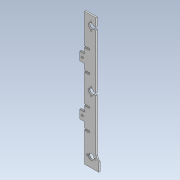
# Autodesk Inventor part: chassis_1_1_3
Saved by Autodesk Inventor 2022 (Build 260153000, 153)
## iProperties
Created: 2023-04-21
Part Number: chassis_1_1_3
Material: 一般
Document SubType Name: Modeling
Designer: JOU
Density: 1 g/cm^3
Appearance: 預設
Author: JOU
Autodesk Inventor part; units mm, degrees
ref_plane "YZ Plane" through (0, 0, 0) normal (1, 0, 0) x (0, 1, 0)
ref_plane "XZ Plane" through (0, 0, 0) normal (0, 1, 0) x (-1, 0, 0)
ref_plane "XY Plane" through (0, 0, 0) normal (0, 0, 1) x (1, 0, 0)
sketch "草圖1" plane through (0, 0, 0) normal (0, 0, 1) x (1, 0, 0)
  line L0 (-6, 142.5) -> (-10.5456, 142.5)
  arc A0 (-10.5456, 147.5) -> (-10.5456, 142.5) centre (-16, 145) ccw
  line L1 (-10.5456, 147.5) -> (-6, 147.5)
  circle A1 centre (-16, 153.5) radius 1.5
  circle A2 centre (-16, 136.5) radius 1.5
  circle A3 centre (-16, 275) radius 1.5
  circle A4 centre (-16, 258) radius 1.5
  circle A5 centre (-16, 23.5) radius 6
  circle A6 centre (-24.5, 23.5) radius 1.5
  circle A7 centre (-7.5, 23.5) radius 1.5
  line L2 (-6, 3) -> (-6, 16)
  line L3 (-6, 31) -> (-6, 142.5)
  arc A8 (-6, 16) -> (-6, 31) centre (-16, 23.5) ccw
  line L4 (-28.5, 3) -> (-28.5, 287)
  arc A9 (-10.546, 269.0008) -> (-10.546, 263.9992) centre (-16, 266.5) ccw
  line L5 (-28.5, 3) -> (-6, 3)
  line L6 (-6, 287) -> (-28.5, 287)
  line L7 (-6, 269.0008) -> (-10.546, 269.0008)
  line L8 (-10.546, 263.9992) -> (-6, 263.9992)
  line L9 (-6, 147.5) -> (-6, 263.9992)
  line L10 (-6, 269.0008) -> (-6, 287)
  circle A10 centre (-16, 23.5) radius 12.5 construction
  line L11 (-6, 72.05) -> (-6, 75)
  line L12 (-19.5, 70) -> (-19.5, 67.05)
  line L13 (-19.5, 112.05) -> (-19.5, 115)
  line L14 (-6, 110) -> (-6, 107.05)
  line L15 (-6, 182.95) -> (-6, 180)
  line L16 (-6, 217.95) -> (-6, 215)
  line L17 (-19.5, 67.05) -> (-28.5, 67.05)
  line L18 (-28.5, 67.05) -> (-28.5, 70)
  line L19 (-28.5, 70) -> (-19.5, 70)
  line L20 (-19.5, 70) -> (-19.5, 67.05)
  line L21 (-19.5, 112.05) -> (-28.5, 112.05)
  line L22 (-28.5, 112.05) -> (-28.5, 115)
  line L23 (-28.5, 115) -> (-19.5, 115)
  line L24 (-19.5, 115) -> (-19.5, 112.05)
  line L25 (-19.5, 175) -> (-28.5, 175)
  line L26 (-28.5, 175) -> (-28.5, 177.95)
  line L27 (-28.5, 177.95) -> (-19.5, 177.95)
  line L28 (-19.5, 177.95) -> (-19.5, 175)
  line L29 (-28.5, 220) -> (-19.5, 220)
  line L30 (-19.5, 220) -> (-19.5, 222.95)
  line L31 (-19.5, 222.95) -> (-28.5, 222.95)
  line L32 (-28.5, 222.95) -> (-28.5, 220)
  line L33 (-6, 3) -> (-3.5, 3)
  line L34 (-3.5, 3) -> (-3.5, 23.5)
  line L35 (-3.5, 23.5) -> (-6, 23.5)
  line L36 (-6, 23.5) -> (-6, 3)
  line L37 (-3.5, 3) -> (0, 3)
  line L38 (0, 3) -> (0, 23.5)
  line L39 (0, 23.5) -> (-3.5, 23.5)
  line L40 (-3.5, 23.5) -> (-3.5, 3)
  point P0 (0, 0)
  point P1 (0, 0)
  point P2 (-28.5, 222.95)
  point P3 (-28.5, 220)
  point P4 (-28.5, 175)
  point P5 (-28.5, 112.05)
  point P6 (-28.5, 67.05)
  point P7 (-3.5, 23.5)
  dimension "d0" = 12
  dimension "d3" = 3
  dimension "d4" = 12
  dimension "d5" = 10
  dimension "d6" = 12.5
  dimension "d9" = 8.5
  dimension "d10" = 8.5
  dimension "d12" = 20.5
  dimension "d13" = 4.546
  dimension "d14" = 5.0015
  dimension "d27" = 75
  dimension "d28" = 30
  dimension "d29" = 30
  dimension "d30" = 75
  dimension "d31" = 2.95
  dimension "d32" = 9
  dimension "d33" = 2.95
  dimension "d34" = 2.95
  dimension "d35" = 2.95
  dimension "d58" = 2.5
  dimension "d59" = 3.5
  constraints: 82 end point, 15 parallel, 11 horizontal, 10 centre point, 8 point on line, 7 point on circle, 6 perpendicular, 5 collinear, 5 vertical, 2 coincident, 2 horizontal alignment, 1 equal radius, 22 other
  measures "d0" diameter of A5
  measures "d3" diameter of A6
  measures "d4" diameter of A9
  measures "d5" distance from line of L2 A8.centre
  measures "d6" radius of A8
  measures "d9" distance of A8.centre A6.centre
  measures "d10" distance of A8.centre A7.centre
  measures "d12" distance from line of A5.centre L5
  measures "d13" distance of L8.start L8.end
  measures "d14" distance between parallel lines of L8 L7
  measures "d27" distance from line of A0.centre L19
  measures "d28" distance from line of A0.centre L23
  measures "d29" distance from line of L25 A0.centre
  measures "d30" distance from line of A0.centre L29
  measures "d31" distance between parallel lines of L29 L31
  measures "d32" distance of L29.start L29.end
  measures "d33" distance between parallel lines of L25 L27
  measures "d34" distance between parallel lines of L19 L17
  measures "d35" distance between parallel lines of L23 L21
  measures "d58" distance of L2.start L33.end
  measures "d59" distance of L33.end L37.end
extrude "擠出1" add sketch "草圖1" along normal blind 3 contours L3 A8 L35 L36 L2 L5 L4 L17 L12 L19 L21 L13 L23 L25 L28 L27 L29 L30 L31 L6 L10 L7 A9 L8 L9 L1 A0 L0 | L34 L33 L2 A8 | L39 L38 L37 L34 | A8 L36 L35
sketch "草圖2" plane through (0, 0, 0) normal (0, 0, -1) x (-1, 0, 0)
  line L0 (28.5, 287) -> (28.5, 222.95) projected
  line L1 (28.5, 287) -> (30.5, 287)
  line L2 (30.5, 287) -> (30.5, 222.95)
  line L3 (30.5, 220) -> (28.5, 220)
  line L4 (28.5, 220) -> (28.5, 177.95) projected
  line L5 (28.5, 222.95) -> (30.5, 222.95)
  line L6 (30.5, 220) -> (30.5, 177.95)
  line L7 (30.5, 177.95) -> (28.5, 177.95)
  line L8 (28.5, 177.95) -> (28.5, 220)
  line L9 (28.5, 175) -> (28.5, 115) projected
  line L10 (28.5, 175) -> (30.5, 175)
  line L11 (30.5, 175) -> (30.5, 115)
  line L12 (30.5, 115) -> (28.5, 115)
  line L13 (28.5, 115) -> (28.5, 175)
  line L14 (28.5, 112.05) -> (28.5, 70) projected
  line L15 (28.5, 112.05) -> (30.5, 112.05)
  line L16 (30.5, 112.05) -> (30.5, 70)
  line L17 (30.5, 70) -> (28.5, 70)
  line L18 (28.5, 70) -> (28.5, 112.05)
  line L19 (19.5, 67.05) -> (28.5, 67.05) projected
  line L20 (28.5, 67.05) -> (30.5, 67.05)
  line L21 (30.5, 67.05) -> (30.5, 3)
  line L22 (30.5, 3) -> (28.5, 3)
  line L23 (28.5, 3) -> (28.5, 67.05)
  line L24 (28.5, 177.95) -> (19.5, 177.95) projected
  line L25 (28.5, 115) -> (19.5, 115) projected
  line L26 (28.5, 70) -> (19.5, 70) projected
  line L27 (28.5, 222.95) -> (19.5, 222.95) projected
  line L28 (19.5, 220) -> (28.5, 220) projected
  line L29 (28.5, 220) -> (28.5, 220)
  line L30 (28.5, 222.95) -> (28.5, 287)
  line L31 (28.5, 3) -> (0, 3) projected
  point P0 (0, 0)
  point P1 (19.5, 75)
  point P2 (28.5, 217.95)
  point P3 (28.5, 70)
  point P4 (3.5, 3)
  dimension "d36" = 2
  constraints: 44 end point, 11 parallel, 6 collinear, 6 horizontal, 5 perpendicular, 2 point on line, 1 other
  measures "d36" distance between parallel lines of L23 L21
extrude "擠出2" add sketch "草圖2" against normal up to surface (3 mm away)
sketch "草圖3" plane through (0, 0, 0) normal (0, 0, -1) x (-1, 0, 0)
  line L0 (40.5, 208) -> (30.5, 208)
  line L1 (30.5, 208) -> (30.5, 190)
  line L2 (30.5, 190) -> (40.5, 190)
  line L3 (40.5, 190) -> (40.5, 208)
  line L4 (40.5, 100) -> (30.5, 100)
  line L5 (30.5, 100) -> (30.5, 82)
  line L6 (30.5, 82) -> (40.5, 82)
  line L7 (40.5, 82) -> (40.5, 100)
  line L8 (30.5, 70) -> (30.5, 112.05) projected
  line L9 (30.5, 177.95) -> (30.5, 220) projected
  line L10 (19.5, 220) -> (28.5, 220) projected
  point P0 (0, 0)
  point P1 (30.5, 215)
  dimension "d39" = 18
  dimension "d40" = 18
  dimension "d41" = 10
  dimension "d42" = 10
  dimension "d43" = 12
  dimension "d44" = 90
  constraints: 16 end point, 4 parallel, 2 collinear, 2 horizontal, 2 perpendicular, 1 other
  measures "d39" distance of L6.end L4.start
  measures "d40" distance between parallel lines of L0 L2
  measures "d41" distance between parallel lines of L5 L7
  measures "d42" distance between parallel lines of L1 L3
  measures "d44" distance between parallel lines of L4 L2
extrude "擠出3" add sketch "草圖3" against normal up to surface (3 mm away)
sketch "草圖5" plane through (0, 0, 3) normal (0, 0, 1) x (1, 0, 0)
  line L0 (-36.4, 92.5) -> (-33.5, 92.5)
  line L1 (-33.5, 92.5) -> (-33.5, 89.5)
  line L2 (-33.5, 89.5) -> (-36.4, 89.5)
  line L3 (-36.4, 89.5) -> (-36.4, 92.5)
  line L4 (-40.5, 82) -> (-40.5, 100) projected
  line L5 (-30.5, 100) -> (-30.5, 112.05) projected
  line L6 (-40.5, 100) -> (-30.5, 100) projected
  line L7 (-36.4, 200.5) -> (-33.5, 200.5)
  line L8 (-33.5, 200.5) -> (-33.5, 197.5)
  line L9 (-33.5, 197.5) -> (-36.4, 197.5)
  line L10 (-36.4, 197.5) -> (-36.4, 200.5)
  line L11 (-40.5, 208) -> (-30.5, 208) projected
  line L12 (-30.5, 208) -> (-30.5, 220) projected
  point P0 (0, 0)
  dimension "d47" = 2.9
  dimension "d48" = 3
  dimension "d50" = 3
  dimension "d51" = 7.5
  dimension "d52" = 2.9
  dimension "d53" = 3
  dimension "d54" = 7.5
  dimension "d55" = 3
  constraints: 16 end point, 4 parallel, 2 horizontal, 2 perpendicular
  measures "d47" distance of L0.start L0.end
  measures "d48" distance of L0.end L1.end
  measures "d50" distance between parallel lines of L5 L1
  measures "d51" distance between parallel lines of L6 L0
  measures "d52" distance of L7.start L7.end
  measures "d53" distance of L7.end L8.end
  measures "d54" distance between parallel lines of L11 L7
  measures "d55" distance between parallel lines of L12 L8
extrude "擠出4" cut sketch "草圖5" against normal up to surface (3 mm away)
fillet "圓角1" radius 2 2 edges at (0, 23.5, 1.5) (-3.5, 23.5, 1.5)
